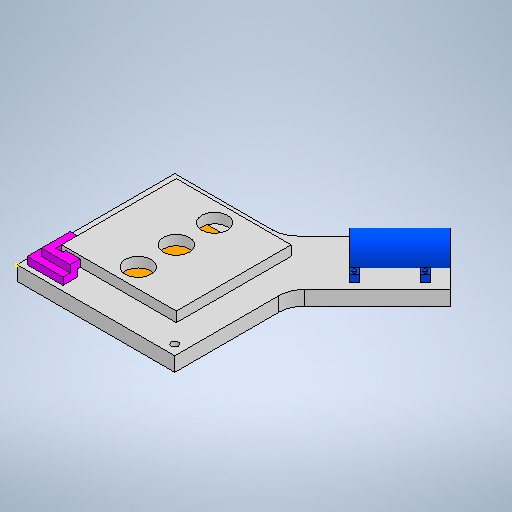
# Autodesk Inventor part: Součást1
Saved by Autodesk Inventor 2025 (Build 290162000, 162)
## iProperties
Created: 2025-05-08
Part Number: Součást1
Material: Všeobecné
Document SubType Name: Modeling
Designer: zdene
Mass: 224.992 g
Surface Area: 525.203 cm^2
Volume: 224.992 cm^3
Density: 1 g/cm^3
Appearance: Výchozí
Author: zdene
Autodesk Inventor part; units mm, degrees
ref_plane "YZ Plane" through (0, 0, 0) normal (1, 0, 0) x (0, 1, 0)
ref_plane "XZ Plane" through (0, 0, 0) normal (0, 1, 0) x (-1, 0, 0)
ref_plane "XY Plane" through (0, 0, 0) normal (0, 0, 1) x (1, 0, 0)
sketch "Náčrt1" plane through (0, 0, 0) normal (0, 0, 1) x (1, 0, 0)
  line L0 (0, 0) -> (110, 0)
  line L1 (110, 0) -> (110, 72.5558)
  line L2 (67.945, 110) -> (0, 110)
  line L3 (0, 110) -> (0, 0)
  line L4 (0, 0) -> (268.4899, 0) construction
  line L5 (166.1231, 136.1347) -> (115.2721, 85.2837)
  line L6 (135.1648, 167.093) -> (80.3503, 114.9574)
  line L7 (166.1231, 136.1347) -> (135.1648, 167.093)
  arc A0 (115.2721, 85.2837) -> (110, 72.5558) centre (128, 72.5558) ccw
  arc A1 (67.945, 110) -> (80.3503, 114.9574) centre (67.945, 128) ccw
  constraints: 16 end point, 4 point on circle, 4 tangent, 2 centre point, 2 horizontal, 2 parallel, 1 perpendicular
extrude "Vysunutí1" add sketch "Náčrt1" along normal blind 10
sketch "Náčrt2" plane through (0, 0, 10) normal (0, 0, 1) x (1, 0, 0)
  line L0 (0, 0) -> (110, 0) projected
  line L1 (0, 0) -> (5, 0) construction
  line L2 (3.5355, 3.5355) -> (13.5355, 3.5355)
  line L3 (8.5355, 28.5355) -> (3.5355, 28.5355)
  line L4 (3.5355, 28.5355) -> (3.5355, 3.5355)
  line L5 (3.5355, 3.5355) -> (28.5355, 3.5355)
  line L6 (28.5355, 3.5355) -> (28.5355, 8.5355)
  line L7 (3.5355, 13.5355) -> (3.5355, 3.5355)
  line L8 (13.5355, 28.5355) -> (8.5355, 28.5355)
  line L9 (8.5355, 28.5355) -> (8.5355, 13.5355)
  line L10 (13.5355, 13.5355) -> (13.5355, 18.5355)
  line L11 (28.5355, 13.5355) -> (13.5355, 13.5355)
  line L12 (8.5355, 13.5355) -> (8.5355, 8.5355)
  line L13 (8.5355, 8.5355) -> (28.5355, 8.5355)
  line L14 (28.5355, 8.5355) -> (28.5355, 13.5355)
  line L15 (13.5355, 28.5355) -> (13.5355, 18.5355)
  line L16 (13.5355, 18.5355) -> (8.5355, 18.5355)
  constraints: 32 end point, 5 horizontal, 5 parallel, 4 perpendicular, 1 point on line
extrude "Vysunutí2" add sketch "Náčrt2" along normal blind 5 contours L4 L3 L9 L12 L13 L6 L5 L2
extrude "Vysunutí3" add sketch "Náčrt2" along normal blind 10 contours L13 L12 L9 L16 L10 L11 L14 | L8 L15 L16 L9
sketch "Náčrt5" plane through (13.5355, 13.5355, 10) normal (1, 0, 0) x (0, 0, -1)
  line L0 (-5, -5) -> (-5, 15) projected
  line L1 (-10, 15) -> (-5, 15)
  line L2 (-5, 15) -> (-5, 5)
  line L3 (-5, 5) -> (-10, 5)
  line L4 (-10, 5) -> (-10, 15)
  point P0 (10, -13.5355)
  constraints: 8 end point, 2 parallel, 1 horizontal, 1 midpoint, 1 perpendicular
extrude "Vysunutí4" add sketch "Náčrt5" along normal blind 2
sketch "Náčrt7" plane through (13.5355, 13.5355, 10) normal (0, 1, 0) x (1, 0, 0)
  line L0 (15, -10) -> (0, -10) projected
  line L1 (15, -5) -> (-5, -5) projected
  line L2 (15, -10) -> (5, -10)
  line L3 (5, -10) -> (5, -5)
  line L4 (5, -5) -> (15, -5)
  line L5 (15, -5) -> (15, -10)
  point P0 (-13.5355, 10)
  constraints: 8 end point, 2 parallel, 1 horizontal, 1 midpoint, 1 perpendicular
extrude "Vysunutí5" add sketch "Náčrt7" along normal blind 2
sketch "Náčrt8" plane through (0, 0, 10) normal (0, 0, 1) x (1, 0, 0)
  line L0 (0, 110) -> (0, 0) projected
  line L1 (0, 110) -> (10, 110) construction
  circle A0 centre (7.0711, 102.9289) radius 2.5
  constraints: 2 end point, 1 centre point, 1 horizontal
extrude "Vysunutí6" cut sketch "Náčrt8" against normal blind 20
sketch "Náčrt9" plane through (0, 0, 10) normal (0, 0, 1) x (1, 0, 0)
  line L0 (0, 0) -> (110, 0) projected
  line L1 (110, 0) -> (102.9289, 7.0711)
  line L2 (110, 0) -> (120, 0) construction
  circle A0 centre (102.9289, 7.0711) radius 2.5
  dimension "d36" = 5
  constraints: 4 end point, 1 centre point, 1 coincident, 1 equal length, 1 horizontal
  measures "d36" diameter of A0
extrude "Vysunutí7" cut sketch "Náčrt9" against normal blind 20
sketch "Náčrt13" plane through (135.1648, 167.093, 0) normal (0.7071, 0.7071, 0) x (-0.7071, 0.7071, 0)
  line L0 (-22.5767, 0) -> (-22.5767, 10) projected
  line L1 (-22.5767, 15) -> (-22.5767, 20) projected
  line L2 (-22.5767, 20) -> (-36.7188, 20) projected
  line L3 (55.2051, 10) -> (-22.5767, 10) projected
  circle A0 centre (-22.5767, 20) radius 10
  dimension "d43" = 10
  constraints: 1 coincident, 1 vertical alignment, 2 other
  measures "d43" distance of L0.end L1.end
extrude "Vysunutí8" add sketch "Náčrt13" against normal blind 50
sketch "Náčrt14" plane through (151.1289, 151.1289, 20) normal (0.7071, 0.7071, 0) x (-0.7071, 0.7071, 0)
  line L0 (0, 0) -> (-14.1421, 0) projected
  circle A0 centre (0, 0) radius 5
  line L1 (0, -5) -> (14.1421, -5) projected
  point P0 (0, -20)
  constraints: 1 horizontal, 1 vertical alignment, 1 other
extrude "Vysunutí9" cut sketch "Náčrt14" against normal blind 50
sketch "Náčrt15" plane through (0, 0, 10) normal (0, 0, 1) x (1, 0, 0)
  line L0 (108.7025, 122.8446) -> (122.8446, 108.7025) projected
  line L1 (122.8446, 108.7025) -> (126.3801, 105.1669)
  line L2 (115.2721, 85.2837) -> (166.1231, 136.1347) projected
  line L3 (126.3801, 105.1669) -> (129.9157, 108.7025)
  line L4 (129.9157, 108.7025) -> (108.7025, 129.9157)
  line L5 (112.238, 126.3801) -> (108.7025, 129.9157)
  line L6 (105.1669, 126.3801) -> (108.7025, 129.9157)
  line L7 (105.1669, 126.3801) -> (122.8446, 108.7025)
  point P0 (0, 0)
  point P1 (115.7735, 115.7735)
  dimension "d48" = 5
  constraints: 12 end point, 4 perpendicular, 1 collinear, 1 point on line
  measures "d48" distance of L0.end L1.end
extrude "Vysunutí10" add sketch "Náčrt15" along normal blind 4.5
sketch "Náčrt16" plane through (0, 0, 10) normal (0, 0, 1) x (1, 0, 0)
  line L0 (119.3091, 119.3091) -> (129.9157, 108.7025) projected
  line L1 (151.1289, 136.9867) -> (154.6644, 133.4512)
  line L2 (154.6644, 133.4512) -> (151.1289, 129.9157)
  line L3 (151.1289, 129.9157) -> (133.4512, 147.5933)
  line L4 (135.1648, 167.093) -> (80.3503, 114.9574) projected
  line L5 (133.4512, 154.6644) -> (151.1289, 136.9867)
  line L6 (144.0578, 158.1999) -> (108.7025, 122.8446) projected
  line L7 (133.4512, 147.5933) -> (129.9157, 151.1289)
  line L8 (129.9157, 151.1289) -> (133.4512, 154.6644)
  point P0 (0, 0)
  constraints: 12 end point, 2 perpendicular, 1 collinear, 1 point on line
extrude "Vysunutí11" add sketch "Náčrt16" along normal blind 4.5
sketch "Náčrt17" plane through (0, 0, 14.5) normal (0, 0, 1) x (1, 0, 0)
  line L0 (108.7025, 129.9157) -> (105.1669, 126.3801) projected
  circle A0 centre (108.7025, 126.3801) radius 1.25
  point P0 (0, 0)
  constraints: 1 centre point
extrude "Vysunutí12" add sketch "Náčrt17" along normal blind 1
sketch "Náčrt18" plane through (0, 0, 14.5) normal (0, 0, 1) x (1, 0, 0)
  line L0 (140.5223, 140.5223) -> (129.9157, 151.1289) projected
  line L1 (129.9157, 151.1289) -> (133.4512, 154.6644) projected
  circle A0 centre (133.4512, 151.1289) radius 1.25
  point P0 (0, 0)
  constraints: 1 centre point
extrude "Vysunutí13" add sketch "Náčrt18" along normal blind 1
sketch "Náčrt19" plane through (0, 0, 14.5) normal (0, 0, 1) x (1, 0, 0)
  line L0 (154.6644, 133.4512) -> (151.1289, 129.9157) projected
  circle A0 centre (151.1289, 133.4512) radius 1.25
  point P0 (0, 0)
  constraints: 1 centre point
extrude "Vysunutí14" add sketch "Náčrt19" along normal blind 1
sketch "Náčrt20" plane through (0, 0, 14.5) normal (0, 0, 1) x (1, 0, 0)
  line L0 (119.3091, 119.3091) -> (129.9157, 108.7025) projected
  line L1 (126.3801, 105.1669) -> (105.1669, 126.3801) projected
  circle A0 centre (126.3801, 108.7025) radius 1.25
  point P0 (0, 0)
  constraints: 1 centre point
extrude "Vysunutí15" add sketch "Náčrt20" along normal blind 1
sketch "Náčrt22" plane through (0, 0, 15) normal (0, 0, 1) x (1, 0, 0)
  line L0 (18.5355, 13.5355) -> (18.5355, 15.5355) projected
  line L1 (18.5355, 15.5355) -> (15.5355, 15.5355)
  line L2 (15.5355, 15.5355) -> (95.5355, 15.5355)
  line L3 (95.5355, 15.5355) -> (95.5355, 95.5355)
  line L4 (95.5355, 95.5355) -> (15.5355, 95.5355)
  line L5 (15.5355, 95.5355) -> (15.5355, 15.5355)
  point P0 (0, 0)
  dimension "d63" = 80
  dimension "d64" = 80
  constraints: 10 end point, 2 horizontal, 2 parallel, 1 perpendicular
  measures "d63" distance of L4.end L3.end
  measures "d64" distance of L3.end L2.end
extrude "Vysunutí16" add sketch "Náčrt22" along normal blind 7
sketch "Náčrt25" plane through (0, 0, 10) normal (0, 0, 1) x (1, 0, 0)
  line L0 (95.5355, 95.5355) -> (95.5355, 85.5355)
  line L1 (95.5355, 15.5355) -> (95.5355, 95.5355) projected
  line L2 (15.5355, 95.5355) -> (15.5355, 15.5355) projected
  line L3 (85.5355, 85.5355) -> (25.5355, 85.5355)
  line L4 (95.5355, 85.5355) -> (85.5355, 85.5355)
  line L5 (85.5355, 85.5355) -> (85.5355, 25.5355)
  line L6 (85.5355, 25.5355) -> (25.5355, 25.5355)
  line L7 (25.5355, 25.5355) -> (25.5355, 85.5355)
  point P0 (0, 0)
  constraints: 12 end point, 3 perpendicular, 1 horizontal, 1 point on line
extrude "Vysunutí17" add sketch "Náčrt25" along normal blind 5
sketch "Náčrt26" plane through (0, 0, 22) normal (0, 0, 1) x (1, 0, 0)
  line L0 (95.5355, 95.5355) -> (15.5355, 95.5355) projected
  line L1 (28.5355, 15.5355) -> (95.5355, 15.5355) projected
  circle A0 centre (55.5355, 82.2055) radius 9
  circle A1 centre (55.5355, 55.5455) radius 9
  circle A2 centre (55.5355, 28.8655) radius 9
  point P0 (0, 0)
  constraints: 3 centre point
extrude "Vysunutí18" cut sketch "Náčrt26" against normal blind 7
sketch "Náčrt29" plane through (0, 0, 10) normal (0, 0, 1) x (1, 0, 0)
  point P0 (0, 0)
